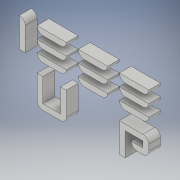
# Autodesk Inventor part: ieee
Saved by Autodesk Inventor 2018 (Build 220112000, 112)
## iProperties
Created: 2017-04-27
Part Number: ieee
Material: Generic
Document SubType Name: Modeling
Designer: visual15
Density: 1 g/cm^3
Appearance: Default
Author: visual15
Autodesk Inventor part; units mm, degrees
ref_plane "YZ Plane" through (0, 0, 0) normal (1, 0, 0) x (0, 1, 0)
ref_plane "XZ Plane" through (0, 0, 0) normal (0, 1, 0) x (-1, 0, 0)
ref_plane "XY Plane" through (0, 0, 0) normal (0, 0, 1) x (1, 0, 0)
sketch "Sketch5" plane through (0, 0, 0) normal (0, 0, 1) x (1, 0, 0)
  line L0 (0, 0) -> (2, 0)
  line L1 (2, 0) -> (2, 8)
  line L2 (0, 10) -> (0, 10)
  line L3 (0, 10) -> (0, 0)
  line L4 (6, 10) -> (16, 10)
  line L5 (16, 10) -> (16, 10)
  line L6 (14, 8) -> (8, 8)
  line L7 (6, 10) -> (6, 10)
  line L8 (6, 6) -> (16, 6)
  line L9 (16, 6) -> (16, 6)
  line L10 (14, 4) -> (8, 4)
  line L11 (6, 6) -> (6, 6)
  line L12 (6, 2) -> (16, 2)
  line L13 (16, 2) -> (16, 2)
  line L14 (14, 0) -> (8, 0)
  line L15 (6, 2) -> (6, 2)
  line L16 (20, 10) -> (30, 10)
  line L17 (30, 10) -> (30, 10)
  line L18 (28, 8) -> (22, 8)
  line L19 (20, 10) -> (20, 10)
  line L20 (20, 6) -> (30, 6)
  line L21 (30, 6) -> (30, 6)
  line L22 (28, 4) -> (22, 4)
  line L23 (20, 6) -> (20, 6)
  line L24 (20, 2) -> (30, 2)
  line L25 (30, 2) -> (30, 2)
  line L26 (28, 0) -> (22, 0)
  line L27 (20, 2) -> (20, 2)
  line L28 (34, 10) -> (44, 10)
  line L29 (44, 10) -> (44, 10)
  line L30 (42, 8) -> (36, 8)
  line L31 (34, 10) -> (34, 10)
  line L32 (34, 6) -> (44, 6)
  line L33 (44, 6) -> (44, 6)
  line L34 (42, 4) -> (36, 4)
  line L35 (34, 6) -> (34, 6)
  line L36 (34, 2) -> (44, 2)
  line L37 (44, 2) -> (44, 2)
  line L38 (42, 0) -> (36, 0)
  line L39 (34, 2) -> (34, 2)
  arc A0 (2, 8) -> (0, 10) centre (0, 8) ccw
  arc A1 (6, 10) -> (8, 8) centre (8, 10) ccw
  arc A2 (6, 6) -> (8, 4) centre (8, 6) ccw
  arc A3 (6, 2) -> (8, 0) centre (8, 2) ccw
  arc A4 (14, 0) -> (16, 2) centre (14, 2) ccw
  arc A5 (14, 4) -> (16, 6) centre (14, 6) ccw
  arc A6 (14, 8) -> (16, 10) centre (14, 10) ccw
  arc A7 (20, 10) -> (22, 8) centre (22, 10) ccw
  arc A8 (20, 6) -> (22, 4) centre (22, 6) ccw
  arc A9 (20, 2) -> (22, 0) centre (22, 2) ccw
  arc A10 (28, 0) -> (30, 2) centre (28, 2) ccw
  arc A11 (28, 4) -> (30, 6) centre (28, 6) ccw
  arc A12 (28, 8) -> (30, 10) centre (28, 10) ccw
  arc A13 (34, 10) -> (36, 8) centre (36, 10) ccw
  arc A14 (34, 6) -> (36, 4) centre (36, 6) ccw
  arc A15 (34, 2) -> (36, 0) centre (36, 2) ccw
  arc A16 (42, 0) -> (44, 2) centre (42, 2) ccw
  arc A17 (42, 4) -> (44, 6) centre (42, 6) ccw
  arc A18 (42, 8) -> (44, 10) centre (42, 10) ccw
  line L40 (6, -4) -> (8, -4)
  line L41 (8, -4) -> (8, -12)
  line L42 (8, -12) -> (14, -12)
  line L43 (14, -12) -> (14, -4)
  line L44 (14, -4) -> (16, -4)
  line L45 (16, -4) -> (16, -12)
  line L46 (14, -14) -> (8, -14)
  line L47 (6, -12) -> (6, -4)
  arc A19 (6, -12) -> (8, -14) centre (8, -12) ccw
  arc A20 (14, -14) -> (16, -12) centre (14, -12) ccw
  line L48 (6, 0) -> (6, 10) construction
  line L49 (20, -14) -> (20, -4)
  line L50 (20, -4) -> (28, -4)
  line L51 (30, -6) -> (30, -8)
  line L52 (20, -14) -> (22, -14)
  line L53 (22, -14) -> (22, -6)
  line L54 (22, -6) -> (28, -6)
  arc A21 (30, -6) -> (28, -4) centre (28, -6) ccw
  line L55 (30, -12) -> (30, -14)
  line L56 (30, -14) -> (28, -14)
  line L57 (20, 10) -> (20, 0) construction
  line L58 (34, -4) -> (34, -14)
  line L59 (34, -4) -> (42, -4)
  line L60 (34, -14) -> (36, -14)
  line L61 (36, -14) -> (36, -6)
  line L62 (36, -6) -> (42, -6)
  line L63 (42, -6) -> (42, -8)
  line L64 (38, -8) -> (42, -8)
  line L65 (38, -8) -> (38, -8)
  line L66 (44, -6) -> (44, -8)
  line L67 (42, -10) -> (40, -10)
  line L68 (34, 10) -> (34, 0) construction
  arc A22 (38, -8) -> (40, -10) centre (40, -8) ccw
  arc A23 (42, -10) -> (44, -8) centre (42, -8) ccw
  arc A24 (44, -6) -> (42, -4) centre (42, -6) ccw
  line L69 (28, -6) -> (28, -8)
  line L70 (30, -8) -> (30, -8)
  line L71 (30, -12) -> (30, -12)
  line L72 (28, -10) -> (28, -10)
  arc A25 (30, -12) -> (28, -10) centre (28, -12) ccw
  line L73 (28, -10) -> (28, -10)
  arc A26 (28, -10) -> (30, -8) centre (28, -8) ccw
  line L74 (28, -8) -> (26, -8)
  line L75 (28, -12) -> (26, -12)
  line L76 (28, -12) -> (28, -14)
  line L77 (24, -10) -> (24, -10)
  arc A27 (26, -8) -> (24, -10) centre (26, -10) ccw
  line L78 (24, -10) -> (24, -10)
  arc A28 (24, -10) -> (26, -12) centre (26, -10) ccw
  point P0 (2, 10)
  point P1 (16, 8)
  point P2 (6, 8)
  point P3 (16, 4)
  point P4 (6, 4)
  point P5 (16, 0)
  point P6 (30, 8)
  point P7 (20, 8)
  point P8 (30, 4)
  point P9 (20, 4)
  point P10 (30, 0)
  point P11 (44, 8)
  point P12 (34, 8)
  point P13 (44, 4)
  point P14 (34, 4)
  point P15 (44, 0)
  point P16 (30, -4)
  point P17 (30, -10)
  point P18 (44, -4)
  point P19 (38, -10)
  point P20 (24, -8)
  dimension "d59" = 2
  dimension "d60" = 10
  dimension "d61" = 10
  dimension "d62" = 2
  dimension "d63" = 10
  dimension "d64" = 2
  dimension "d65" = 10
  dimension "d66" = 2
  dimension "d67" = 4
  dimension "d68" = 2
  dimension "d69" = 10
  dimension "d70" = 2
  dimension "d71" = 4
  dimension "d72" = 10
  dimension "d73" = 2
  dimension "d74" = 10
  dimension "d75" = 2
  dimension "d76" = 10
  dimension "d77" = 2
  dimension "d78" = 4
  dimension "d79" = 10
  dimension "d80" = 2
  dimension "d81" = 10
  dimension "d82" = 2
  dimension "d83" = 2
  dimension "d84" = 4
  dimension "d85" = 2
  dimension "d86" = 2
  dimension "d87" = 2
  dimension "d88" = 2
  dimension "d89" = 10
  dimension "d90" = 10
  dimension "d91" = 6
  dimension "d93" = 2
  dimension "d96" = 10
  dimension "d97" = 2
  dimension "d98" = 2
  dimension "d101" = 2
  dimension "d102" = 2
  dimension "d103" = 2
  dimension "d104" = 2
  dimension "d105" = 2
  dimension "d106" = 10
  dimension "d107" = 6
  dimension "d108" = 2
  dimension "d112" = 2
  dimension "d113" = 2
  dimension "d114" = 4
  dimension "d115" = 2
  dimension "d116" = 2
  dimension "d117" = 4
  dimension "d118" = 2
  dimension "d119" = 2
  constraints: 158 end point, 60 tangent, 58 point on circle, 54 point on line, 29 centre point, 23 collinear, 23 perpendicular, 21 equal radius, 21 horizontal, 20 parallel, 13 vertical
  measures "d59" distance of L2.end point (2, 10)
  measures "d60" distance of point (2, 10) L0.end
  measures "d61" distance of point (16, 8) point (6, 8)
  measures "d62" distance of L4.end point (16, 8)
  measures "d63" distance of point (16, 4) point (6, 4)
  measures "d64" distance of L8.end point (16, 4)
  measures "d65" distance of point (16, 0) L48.start
  measures "d66" distance of L12.end point (16, 0)
  measures "d67" distance between parallel lines of L1 L7
  measures "d68" distance between parallel lines of L8 L6
  measures "d69" distance of point (30, 8) point (20, 8)
  measures "d70" distance of L16.end point (30, 8)
  measures "d71" distance between parallel lines of L5 L19
  measures "d72" distance of point (30, 4) point (20, 4)
  measures "d73" distance of L20.end point (30, 4)
  measures "d74" distance of point (30, 0) L57.end
  measures "d75" distance of L24.end point (30, 0)
  measures "d76" distance of point (44, 8) point (34, 8)
  measures "d77" distance of L28.end point (44, 8)
  measures "d78" distance between parallel lines of L17 L31
  measures "d79" distance of point (44, 4) point (34, 4)
  measures "d80" distance of L32.end point (44, 4)
  measures "d81" distance of point (44, 0) L68.end
  measures "d82" distance of L36.end point (44, 0)
  measures "d83" radius of A0
  measures "d84" distance between parallel lines of L14 L40
  measures "d85" distance between parallel lines of L47 L41
  measures "d86" distance of L43.end L44.end
  measures "d87" distance between parallel lines of L46 L42
  measures "d88" radius of A19
  measures "d89" distance between parallel lines of L46 L40
  measures "d90" distance between parallel lines of L47 L45
  measures "d91" distance of point (30, -4) point (30, -10)
  measures "d93" radius of A21
  measures "d96" distance between parallel lines of L49 L51
  measures "d97" distance between parallel lines of L50 L54
  measures "d98" distance between parallel lines of L49 L53
  measures "d101" distance of L58.end L60.end
  measures "d102" distance between parallel lines of L59 L62
  measures "d103" distance of L64.start point (38, -10)
  measures "d104" distance of L62.end L63.end
  measures "d105" distance between parallel lines of L66 L63
  measures "d106" distance of L58.start point (44, -4)
  measures "d107" distance between parallel lines of L66 L65
  measures "d108" radius of A22
  measures "d112" radius of A25
  measures "d113" radius of A26
  measures "d114" distance of L74.start point (24, -8)
  measures "d115" distance between parallel lines of L54 L74
  measures "d116" distance of point (24, -8) L77.end
  measures "d117" distance between parallel lines of L69 L77
  measures "d118" radius of A27
  measures "d119" radius of A28
extrude "Extrusion3" add sketch "Sketch5" along normal blind 4 contours L3 A0 L1 L0 | L4 A6 L6 A1 | L8 A5 L10 A2 | L12 A4 L14 A3 | L16 A12 L18 A7 | L20 A11 L22 A8 | L24 A10 L26 A9 | L28 A18 L30 A13 | L32 A17 L34 A14 | L36 A16 L38 A15 | L40 L41 L42 L43 L44 L45 A20 L46 A19 L47 | L59 A24 L66 A23 L67 A22 L64 L63 L62 L61 L60 L58
equation "\"d67\" = 2 * d59"
equation "\"d68\" = d59"
equation "\"d71\" = d67"
equation "\"d78\" = d67"
equation "\"d84\" = d67"
equation "\"d85\" = d59"
equation "\"d86\" = d59"
equation "\"d87\" = d59"
equation "\"d89\" = d60"
equation "\"d90\" = d89"
body "Solid3"
